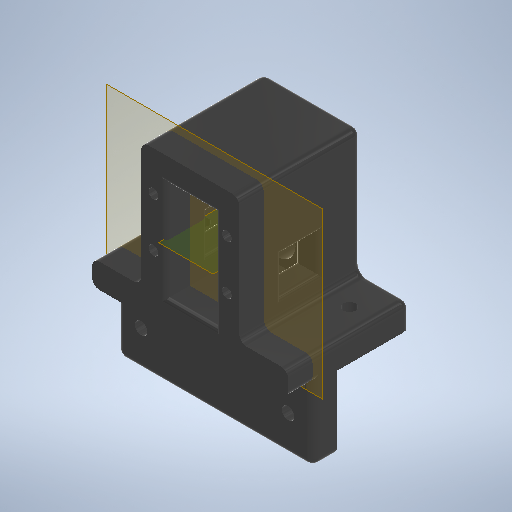
# Autodesk Inventor part: motor_bracket3
Saved by Autodesk Inventor 2026.2 (Build 302298010, 298A)
## iProperties
Created: 2026-04-13
Part Number: motor_bracket3
Material: ABS Plastic
Document SubType Name: Modeling
Designer: chris
Density: 1.06 g/cm^3
Appearance: Smooth - White
Author: chris
Autodesk Inventor part; units mm, degrees
ref_plane "YZ Plane" through (0, 0, 0) normal (1, 0, 0) x (0, 1, 0)
ref_plane "XZ Plane" through (0, 0, 0) normal (0, 1, 0) x (-1, 0, 0)
ref_plane "XY Plane" through (0, 0, 0) normal (0, 0, 1) x (1, 0, 0)
sketch "Sketch1" plane through (0, 0, 0) normal (0, 0, 1) x (1, 0, 0)
  line L0 (-20, -25.05) -> (20, -25.05)
  line L1 (20, -25.05) -> (20, 25.05)
  line L2 (20, 25.05) -> (-20, 25.05)
  line L3 (-20, 25.05) -> (-20, -25.05)
  line L4 (-20, -25.05) -> (20, 25.05) construction
  line L5 (20, -25.05) -> (-20, 25.05) construction
  point P0 (0, 0)
  dimension "d0" = 40
  dimension "d1" = 50.1
  constraints: 12 end point, 2 midpoint, 2 parallel, 1 horizontal, 1 perpendicular
  measures "d0" distance of L2.end L1.end
  measures "d1" distance of L1.end L0.end
extrude "Extrusion1" add sketch "Sketch1" against normal blind 45.5
sketch "Sketch2" plane through (0, 0, 0) normal (0, 0, 1) x (1, 0, 0)
  line L0 (-10.1, -15.05) -> (10.1, -15.05)
  line L1 (10.1, -15.05) -> (10.1, 25.05)
  line L2 (10.1, 25.05) -> (-10.1, 25.05)
  line L3 (-10.1, 25.05) -> (-10.1, -15.05)
  line L4 (-10.1, -15.05) -> (10.1, 25.05) construction
  line L5 (10.1, -15.05) -> (-10.1, 25.05) construction
  line L6 (20, 25.05) -> (-20, 25.05) projected
  point P0 (0, 0)
  point P1 (0, 5)
  dimension "d4" = 20.2
  dimension "d5" = 40.1
  constraints: 12 end point, 2 midpoint, 2 parallel, 1 collinear, 1 horizontal, 1 perpendicular
  measures "d4" distance of L2.end L1.end
  measures "d5" distance of L1.end L0.end
extrude "Extrusion2" cut sketch "Sketch2" against normal blind 35.5
sketch "Sketch3" plane through (0, 0, -35.5) normal (0, 0, 1) x (1, 0, 0)
  circle A0 centre (0, -5.05) radius 7.5
  line L0 (10.1, -15.05) -> (-10.1, -15.05) projected
  point P0 (0, 0)
  dimension "d8" = 15
  dimension "d9" = 10
  constraints: 1 centre point
  measures "d8" diameter of A0
  measures "d9" distance from line of L0 A0.centre
extrude "Extrusion3" cut sketch "Sketch3" against normal blind 6
sketch "Sketch5" plane through (20, -25.05, 0) normal (1, 0, 0) x (0, 0, -1)
  line L0 (17.5, 17.5) -> (32.5, 17.5)
  line L1 (32.5, 17.5) -> (32.5, 32.5)
  line L2 (32.5, 32.5) -> (17.5, 32.5)
  line L3 (17.5, 32.5) -> (17.5, 17.5)
  line L4 (17.5, 17.5) -> (32.5, 32.5) construction
  line L5 (32.5, 17.5) -> (17.5, 32.5) construction
  line L6 (45.5, 50.1) -> (45.5, 0) projected
  line L7 (0, 0) -> (45.5, 0) projected
  point P0 (0, 25.05)
  point P1 (25, 25)
  dimension "d17" = 15
  dimension "d18" = 15
  dimension "d19" = 13
  dimension "d20" = 17.5
  constraints: 12 end point, 2 midpoint, 2 parallel, 1 horizontal, 1 perpendicular
  measures "d17" distance of L2.end L1.end
  measures "d18" distance of L1.end L0.end
  measures "d19" distance between parallel lines of L6 L1
  measures "d20" distance between parallel lines of L7 L0
extrude "Extrusion5" cut sketch "Sketch5" against normal through all
ref_plane "Work Plane1" through (0, 0, -55.5) normal (0, 0, -1) x (-1, 0, 0)
sketch "Sketch11" plane through (0, 0, -55.5) normal (0, 0, -1) x (-1, 0, 0)
  ellipse E0 centre (-7.952, -12.932) end of major axis (-8.818, -13.798) minor radius 1 (-9.07, -13.1556) -> (-8.1756, -14.05) ccw projected
  line L0 (8.1756, -14.05) -> (-8.1756, -14.05) projected
  ellipse E1 centre (7.952, -12.932) end of major axis (8.818, -13.798) minor radius 1 (8.1756, -14.05) -> (9.07, -13.1556) ccw projected
  line L1 (9.07, 23.1556) -> (9.07, -13.1556) projected
  ellipse E2 centre (7.952, 22.932) end of major axis (8.818, 23.798) minor radius 1 (9.07, 23.1556) -> (8.1756, 24.05) ccw projected
  line L2 (-8.1756, 24.05) -> (8.1756, 24.05) projected
  ellipse E3 centre (-7.952, 22.932) end of major axis (-8.818, 23.798) minor radius 1 (-8.1756, 24.05) -> (-9.07, 23.1556) ccw projected
  line L3 (-9.07, -13.1556) -> (-9.07, 23.1556) projected
  circle A0 centre (7.525, 22.55) radius 0.7835 projected
  circle A1 centre (-7.525, 22.55) radius 0.7835 projected
  circle A2 centre (7.525, 7.45) radius 0.7835 projected
  circle A3 centre (-7.525, 7.45) radius 0.7835 projected
  circle A4 centre (7.525, -12.55) radius 0.7835 projected
  circle A5 centre (-7.525, -12.55) radius 0.7835 projected
  circle A6 centre (0, -5.05) radius 6.4 projected
  point P0 (0, 0)
  constraints: 4 other
hole "Hole1" at (-7.525, 7.45, -55.5) at (-7.525, -12.55, -55.5) at (7.525, 7.45, -55.5) at (7.525, -12.55, -55.5) at (-7.525, 22.55, -55.5) at (7.525, 22.55, -55.5) direction (0, 0, 1) diameter 2.1 end through all
ref_plane "Work Plane3" through (0, 0, -55.5) normal (0, 0, -1) x (-1, 0, 0)
sketch "Sketch12" plane through (0, 0, -55.5) normal (0, 0, -1) x (-1, 0, 0)
  circle A0 centre (7.525, 7.45) radius 1.05 projected
  circle A1 centre (7.525, -12.55) radius 1.05 projected
  circle A2 centre (-7.525, -12.55) radius 1.05 projected
  circle A3 centre (-7.525, 7.45) radius 1.05 projected
  circle A4 centre (7.525, 7.45) radius 2
  circle A5 centre (7.525, -12.55) radius 2
  circle A6 centre (-7.525, -12.55) radius 2
  circle A7 centre (-7.525, 7.45) radius 2
  circle A8 centre (-7.525, 22.55) radius 1.05 projected
  circle A9 centre (7.525, 22.55) radius 1.05 projected
  circle A10 centre (-7.525, 22.55) radius 2
  circle A11 centre (7.525, 22.55) radius 2
  point P0 (0, 0)
  dimension "d60" = 4
  dimension "d61" = 4
  dimension "d62" = 4
  dimension "d63" = 4
  dimension "d75" = 4
  dimension "d76" = 4
  constraints: 6 centre point, 6 coincident
  measures "d60" diameter of A4
  measures "d61" diameter of A5
  measures "d62" diameter of A6
  measures "d63" diameter of A7
  measures "d75" diameter of A10
  measures "d76" diameter of A11
extrude "Extrusion11" cut sketch "Sketch12" against normal blind 15 contours A0 | A1 | A2 | A3 | A4 | A5 | A6 | A7 | A10 | A11
sketch "Sketch15" plane through (-20, 25.05, -45.5) normal (0, 1, 0) x (1, 0, 0)
  line L0 (0, -45.5) -> (0, 0)
  line L1 (0, 0) -> (40, 0)
  line L2 (40, 0) -> (40, -45.5)
  line L3 (40, -45.5) -> (30.1, -45.5)
  line L4 (30.1, -45.5) -> (30.1, -10)
  line L5 (30.1, -10) -> (9.9, -10)
  line L6 (9.9, -10) -> (9.9, -45.5)
  line L7 (9.9, -45.5) -> (0, -45.5)
  line L8 (0, 0) -> (40, 0) projected
  line L9 (9.9, -10) -> (30.1, -10) projected
  line L10 (9.9, -45.5) -> (9.9, -10) projected
  line L11 (0, -45.5) -> (0, 0) projected
  line L12 (9.9, -45.5) -> (0, -45.5) projected
  line L13 (30.1, -10) -> (30.1, -45.5) projected
  line L14 (40, -45.5) -> (30.1, -45.5) projected
  line L15 (40, -45.5) -> (40, 0) projected
  point P0 (20, -45.5)
  constraints: 16 end point, 8 collinear, 7 perpendicular, 1 vertical
extrude "Extrusion14" add sketch "Sketch15" along normal blind 1
sketch "Sketch16" plane through (-20, 26.05, -45.5) normal (0, 1, 0) x (1, 0, 0)
  line L0 (-20, -45.5) -> (60, -45.5)
  line L1 (60, -45.5) -> (60, 4.5)
  line L2 (60, 4.5) -> (-20, 4.5)
  line L3 (-20, 4.5) -> (-20, -45.5)
  line L4 (-20, -45.5) -> (60, 4.5) construction
  line L5 (60, -45.5) -> (-20, 4.5) construction
  line L6 (40, -45.5) -> (40, 0) projected
  line L7 (40, 0) -> (0, 0) projected
  line L8 (0, 0) -> (0, -45.5) projected
  line L9 (30.1, -45.5) -> (9.9, -45.5) projected
  point P0 (20, -45.5)
  point P1 (20, -20.5)
  point P2 (20, -45.5)
  dimension "d81" = 50
  dimension "d82" = 80
  constraints: 12 end point, 3 midpoint, 2 parallel, 1 collinear, 1 horizontal, 1 perpendicular, 1 vertical alignment
  measures "d81" distance of L0.end L1.end
  measures "d82" distance of L1.end L2.end
extrude "Extrusion15" add sketch "Sketch16" along normal blind 10
sketch "Sketch17" plane through (0, -5.05, -41.5) normal (0, 0, 1) x (1, 0, 0)
  circle A0 centre (0, 0) radius 7.5 projected
  point P0 (0, 5.05)
extrude "Extrusion16" cut sketch "Sketch17" against normal through all
sketch "Sketch18" plane through (-20, 36.05, -45.5) normal (0, 1, 0) x (1, 0, 0)
  circle A0 centre (50, -10.5) radius 2.55
  circle A1 centre (-10, -10.5) radius 2.55
  line L0 (60, 4.5) -> (-20, 4.5) projected
  line L1 (60, -45.5) -> (60, 4.5) projected
  point P0 (20, -45.5)
  dimension "d85" = 5.1
  dimension "d86" = 5.1
  dimension "d87" = 15
  dimension "d89" = 60
  dimension "d90" = 10
  constraints: 2 centre point, 1 horizontal alignment
  measures "d85" diameter of A1
  measures "d86" diameter of A0
  measures "d87" distance from line of L0 A1.centre
  measures "d89" distance of A0.centre A1.centre
  measures "d90" distance from line of L1 A0.centre
extrude "Extrusion17" cut sketch "Sketch18" against normal blind 10
sketch "Sketch19" plane through (-20, 36.05, -45.5) normal (0, 1, 0) x (1, 0, 0)
  line L0 (-20, -35.5) -> (60, -35.5)
  line L1 (60, -35.5) -> (60, -25.5)
  line L2 (60, -25.5) -> (-20, -25.5)
  line L3 (-20, -25.5) -> (-20, -35.5)
  line L4 (-20, -35.5) -> (60, -25.5) construction
  line L5 (60, -35.5) -> (-20, -25.5) construction
  line L6 (60, 4.5) -> (-20, 4.5) projected
  line L7 (-20, 4.5) -> (-20, -45.5) projected
  line L8 (60, -45.5) -> (60, 4.5) projected
  circle A0 centre (50, -10.5) radius 2.55 projected
  point P0 (20, -45.5)
  point P1 (20, -30.5)
  dimension "d94" = 10
  dimension "d97" = 15
  constraints: 12 end point, 2 collinear, 2 midpoint, 2 parallel, 1 horizontal, 1 perpendicular
  measures "d94" distance of L0.end L1.end
  measures "d97" distance from line of L2 A0.centre
extrude "Extrusion18" add sketch "Sketch19" along normal blind 30 contours L3 L2 L1 L0
sketch "Sketch20" plane through (0, 0, -45.5) normal (0, 0, -1) x (-1, 0, 0)
  circle A0 centre (0, -5.05) radius 7.5 projected
  circle A1 centre (7.525, 7.45) radius 2 projected
  circle A2 centre (-7.525, 7.45) radius 2 projected
  circle A3 centre (7.525, 22.55) radius 2 projected
  circle A4 centre (7.525, -12.55) radius 2 projected
  circle A5 centre (-7.525, -12.55) radius 2 projected
  circle A6 centre (-7.525, 22.55) radius 2 projected
  line L0 (-20, -25.05) -> (-20, 26.05) projected
  line L1 (-20, -25.05) -> (20, -25.05) projected
  line L2 (20, -25.05) -> (20, 26.05) projected
  line L3 (-20, 26.05) -> (20, 26.05) projected
  point P0 (0, 0)
extrude "Extrusion19" add sketch "Sketch20" along normal up to surface (4.5 mm away)
sketch "Sketch21" plane through (-40, 36.05, -10) normal (0, 0, 1) x (1, 0, 0)
  circle A0 centre (70, 15) radius 2.55
  circle A1 centre (10, 15) radius 2.55
  line L0 (80, 0) -> (80, 30) projected
  line L1 (80, 0) -> (0, 0) projected
  point P0 (40, -36.05)
  dimension "d100" = 5.1
  dimension "d101" = 5.1
  dimension "d102" = 60
  dimension "d103" = 10
  dimension "d104" = 15
  constraints: 2 centre point, 1 horizontal alignment
  measures "d100" diameter of A0
  measures "d101" diameter of A1
  measures "d102" distance of A0.centre A1.centre
  measures "d103" distance from line of L0 A0.centre
  measures "d104" distance from line of L1 A0.centre
extrude "Extrusion20" cut sketch "Sketch21" against normal blind 10
sketch "Sketch22" plane through (0, 0, 0) normal (0, 0, 1) x (1, 0, 0)
  circle A0 centre (15, -0.05) radius 2
  circle A1 centre (-15, 19.95) radius 2
  circle A2 centre (-15, -0.05) radius 2
  circle A3 centre (15, 19.95) radius 2
  circle A4 centre (-15, -20.05) radius 2
  circle A5 centre (15, -20.05) radius 2
  line L0 (-20, -25.05) -> (20, -25.05) projected
  line L1 (20, -25.05) -> (20, 26.05) projected
  line L2 (-20, 26.05) -> (-20, -25.05) projected
  point P0 (0, 0)
  dimension "d107" = 4
  dimension "d108" = 4
  dimension "d109" = 4
  dimension "d110" = 4
  dimension "d111" = 4
  dimension "d112" = 4
  dimension "d113" = 5
  dimension "d114" = 5
  dimension "d115" = 5
  dimension "d116" = 5
  dimension "d117" = 5
  dimension "d118" = 5
  dimension "d119" = 5
  dimension "d120" = 5
  dimension "d121" = 25
  dimension "d122" = 45
  dimension "d123" = 25
  dimension "d124" = 45
  constraints: 6 centre point
  measures "d107" diameter of A0
  measures "d108" diameter of A1
  measures "d109" diameter of A2
  measures "d110" diameter of A3
  measures "d111" diameter of A4
  measures "d112" diameter of A5
  measures "d113" distance from line of L0 A4.centre
  measures "d114" distance from line of L0 A5.centre
  measures "d115" distance from line of L1 A0.centre
  measures "d116" distance from line of L1 A3.centre
  measures "d117" distance from line of L2 A2.centre
  measures "d118" distance from line of L2 A1.centre
  measures "d119" distance from line of L2 A4.centre
  measures "d120" distance from line of L1 A5.centre
  measures "d121" distance from line of L0 A0.centre
  measures "d122" distance from line of L0 A3.centre
  measures "d123" distance from line of L0 A2.centre
  measures "d124" distance from line of L0 A1.centre
extrude "Extrusion21" cut sketch "Sketch22" against normal blind 15
ref_plane "Work Plane4" through (0, 0, -10) normal (0, 0, 1) x (1, 0, 0)
ref_plane "Work Plane5" through (-20, 5.5, -45.5) normal (0, -1, 0) x (1, 0, 0)
mirror "Mirror2" about plane through (-20, 5.5, -45.5) normal (0, -1, 0) of "Extrusion15", "Extrusion17", "Extrusion18", "Extrusion20"
sketch "Sketch24" plane through (-40, 26.05, -50) normal (-1, 0, 0) x (0, 0, 1)
  line L0 (50, -10) -> (30, -10) projected
  line L1 (50, 0) -> (50, -10) projected
  line L2 (50, 0) -> (50, 10) projected
  line L3 (40, 10) -> (50, 10) projected
  line L4 (40, 10) -> (40, 40) projected
  line L5 (30, 40) -> (40, 40) projected
  line L6 (30, 10) -> (30, 40) projected
  line L7 (0, 10) -> (30, 10) projected
  line L8 (0, 0) -> (0, 10) projected
  line L9 (0, 0) -> (50, 0) projected
  line L10 (30, -10) -> (30, 0) projected
  point P0 (50, -26.05)
extrude "Extrusion23" cut sketch "Sketch24" against normal up to surface (20 mm away)
mirror "Mirror3" about plane through (0, 0, 0) normal (1, 0, 0) of "Extrusion23"
sketch "Sketch25" plane through (-20, 66.05, -45.5) normal (0, 1, 0) x (1, 0, 0)
  line L0 (40, -35.5) -> (40, -25.5) projected
  line L1 (40, -25.5) -> (0, -25.5) projected
  line L2 (0, -25.5) -> (0, -35.5) projected
  line L3 (0, -35.5) -> (40, -35.5) projected
  point P0 (20, -45.5)
extrude "Extrusion24" cut sketch "Sketch25" against normal up to surface (30 mm away)
fillet "Fillet3" radius 3 20 edges at (40, -15.05, -25) (-40, -15.05, -25) (-40, -40.05, -10) (0, -55.05, -10) (40, -40.05, -10) (40, -25.05, -5) (-40, -25.05, -5) (-40, -20.05, -50) (40, -20.05, -50) (30, -15.05, -50) (-30, -15.05, -50) (-20, 10.5, -50) (0, 36.05, -50) (20, 10.5, -50) (20, 36.05, -25) (-20, 36.05, -25) (-20, -15.05, -25) (20, -15.05, -25) (40, -55.05, -15) (-40, -55.05, -15)
fillet "Fillet4" radius 2 20 edges at (20, -0.05, -17.5) (20, -7.55, -25) (20, -0.05, -32.5) (20, 7.45, -25) (10.1, 5.5, 0) (0, 26.05, 0) (-10.1, 5.5, 0) (0, -15.05, 0) (10.1, -0.05, -32.5) (10.1, 7.45, -25) (10.1, -0.05, -17.5) (10.1, -7.55, -25) (-10.1, -0.05, -32.5) (-10.1, -7.55, -25) (-10.1, -0.05, -17.5) (-10.1, 7.45, -25) (-20, -0.05, -32.5) (-20, 7.45, -25) (-20, -7.55, -25) (-20, -0.05, -17.5)
body "Solid1"
